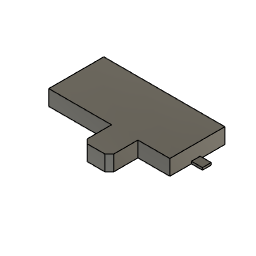
G-Switch_MK-11C04-G013 (Autodesk Fusion 360 design; units mm, degrees)
Autodesk Fusion 360 part; units mm, degrees
sketch "Sketch1" plane through (0, 0, 0) normal (0, 0, 1) x (1, 0, 0)
  line L0 (5.5, 0) -> (5.5, 2.5)
  line L1 (5.5, 2.5) -> (0, 2.5)
  line L2 (0, 2.5) -> (0, 0)
  line L3 (2.75, 2.5) -> (2.75, 0) construction
  line L4 (4.05, 0) -> (4.05, -1.1)
  line L5 (3.85, -1.3) -> (3.05, -1.3)
  line L6 (2.85, -1.1) -> (2.85, 0)
  line L7 (2.85, -1.1) -> (3.05, -1.3)
  line L8 (4.05, -1.1) -> (3.85, -1.3)
  line L9 (2.05, 2.5) -> (2.05, 0) construction
  line L10 (3.45, 2.5) -> (3.45, 0) construction
  line L11 (3.45, -1.3) -> (3.45, 0) construction
  line L12 (0, 1.25) -> (5.5, 1.25) construction
  line L13 (1.25, 2.5) -> (1.25, 0) construction
  line L14 (4.25, 2.5) -> (4.25, 0) construction
  circle A0 centre (1.25, 1.25) radius 0.35
  circle A1 centre (4.25, 1.25) radius 0.35
  line L15 (0, 1.18) -> (5.5, 1.18) construction
  line L16 (-0.5, 1.38) -> (0, 1.38)
  line L17 (0, 1.38) -> (0, 0.98)
  line L18 (0, 0.98) -> (-0.5, 0.98)
  line L19 (-0.5, 0.98) -> (-0.5, 1.38)
  line L20 (5.5, 0.98) -> (5.5, 1.38)
  line L21 (5.5, 1.38) -> (6, 1.38)
  line L22 (6, 1.38) -> (6, 0.98)
  line L23 (6, 0.98) -> (5.5, 0.98)
  line L24 (0, 0) -> (2.85, 0)
  line L25 (4.05, 0) -> (5.5, 0)
  line L26 (2.55, 2.5) -> (2.95, 2.5)
  line L27 (2.95, 2.5) -> (2.95, 3)
  line L28 (2.95, 3) -> (2.55, 3)
  line L29 (2.55, 3) -> (2.55, 2.5)
  line L30 (3.55, 2.5) -> (3.95, 2.5)
  line L31 (3.95, 2.5) -> (3.95, 3)
  line L32 (3.95, 3) -> (3.55, 3)
  line L33 (3.55, 3) -> (3.55, 2.5)
  line L34 (1.55, 2.5) -> (1.95, 2.5)
  line L35 (1.95, 2.5) -> (1.95, 3)
  line L36 (1.95, 3) -> (1.55, 3)
  line L37 (1.55, 3) -> (1.55, 2.5)
  point P0 (4.05, -1.3)
  point P1 (2.85, -1.3)
  point P2 (1.25, 1.25)
  point P3 (4.25, 1.25)
  point P4 (0, 1.18)
  point P5 (5.5, 1.18)
  point P6 (0, 1.18)
  point P7 (5.5, 1.18)
  point P8 (2.75, 2.5)
  point P9 (2.75, 2.5)
  point P10 (1.75, 2.5)
  point P11 (3.75, 2.5)
  point P12 (3.75, 2.5)
  point P13 (1.75, 2.5)
  dimension "d1" = 5.5
  dimension "d2" = 2.5
  dimension "d3" = 1.2
  dimension "d4" = 1.3
  dimension "d5" = 0.2
  dimension "d6" = 0.2
  dimension "d7" = 0.2
  dimension "d8" = 0.2
  dimension "d9" = 0.7
  dimension "d10" = -0.7
  dimension "d13" = 1.5
  dimension "d14" = -1.5
  dimension "d15" = 0.7
  dimension "d16" = 0.7
  dimension "d17" = 1.18
  dimension "d18" = 0.5
  dimension "d19" = 0.4
  dimension "d20" = 0.5
  dimension "d21" = 0.4
  dimension "d22" = 0.4
  dimension "d23" = 0.5
  dimension "d24" = 1
  dimension "d25" = 1
  dimension "d26" = 0.4
  dimension "d27" = 0.5
  dimension "d28" = 0.4
  dimension "d29" = 0.5
  constraint horizontal L24
  constraint vertical L0
  constraint horizontal L1
  constraint vertical L2
  constraint coincident L2.end L24.start
  constraint midpoint L1 P9
  constraint vertical L4
  constraint horizontal L5
  constraint vertical L6
  constraint coincident P1 L6
  constraint coincident P1 L5
  constraint coincident P0 L4
  constraint coincident P0 L5
  constraint midpoint L5 L11.start
  constraint midpoint L2 L12.start
  constraint midpoint L0 L12.end
  constraint coincident L13 P2
  constraint coincident L14 P3
  constraint coincident L2 P6
  constraint coincident L0 P7
  constraint perpendicular L0 L15
  constraint midpoint L13 P2
  constraint midpoint L14 P3
  constraint horizontal L16
  constraint vertical L17
  constraint horizontal L18
  constraint vertical L19
  constraint horizontal L21
  constraint vertical L22
  constraint horizontal L23
  constraint vertical L20
  constraint midpoint L17 P6
  constraint midpoint L20 P7
  constraint coincident P6 P4
  constraint coincident P7 P5
  constraint collinear L24 L25
  constraint coincident L3.end L24
  constraint horizontal L26
  constraint vertical L27
  constraint horizontal L28
  constraint vertical L29
  constraint midpoint L26 P9
  constraint coincident P9 P8
  constraint coincident L1 P12
  constraint horizontal L30
  constraint vertical L31
  constraint horizontal L32
  constraint vertical L33
  constraint midpoint P12 L30
  constraint horizontal L34
  constraint vertical L35
  constraint horizontal L36
  constraint vertical L37
  constraint midpoint P13 L34
  measures "d1" distance of L2.end L0.start
  measures "d2" distance of L2.end L1.end
  measures "d3" distance of L6.end L4.start
  measures "d4" distance of L6.end P1
  measures "d5" distance of P1 L6.start
  measures "d6" distance of P1 L5.end
  measures "d7" distance of P0 L4.end
  measures "d8" distance of P0 L5.start
  measures "d15" diameter of A0
  measures "d16" diameter of A1
  measures "d17" distance of L15 L24
  measures "d18" distance of L16.start L16.end
  measures "d19" distance of L16.start L18.end
  measures "d20" distance of L20.end L21.end
  measures "d21" distance of L20.end L20.start
  measures "d22" distance of L26.start L26.end
  measures "d23" distance of L26.start L28.end
  measures "d24" distance of P9 P12
  measures "d25" distance of P9 P13
  measures "d26" distance of L30.start L30.end
  measures "d27" distance of L30.start L32.end
  measures "d28" distance of L34.start L34.end
  measures "d29" distance of L34.start L36.end
extrude "Extrude1" add sketch "Sketch1" along normal blind 0.7 contours L0 L1 L2 L4 L5 L6 L7 L8 L17 L20 L24 L25 L26 L30 L34 | A0 | A1
extrude "Extrude2" add sketch "Sketch1" against normal blind 0.5 contours A0 | A1
chamfer "Chamfer1" distance 0.05 angle 45 2 edges at (3.9237, 1.3766, -0.5) (0.9237, 1.3766, -0.5)
extrude "Extrude3" add sketch "Sketch1" along normal blind 0.1 contours L0 L20 L21 L22 L23 | L1 L30 L31 L32 L33 | L1 L26 L27 L28 L29 | L1 L34 L35 L36 L37 | L2 L16 L17 L18 L19
equation "d6 = d5"
equation "d8 = d7"
